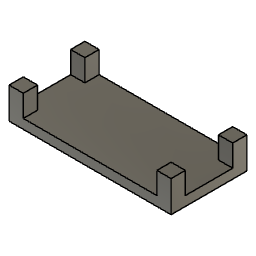
Reservoir Stand (Autodesk Fusion 360 design; units mm, degrees)
Autodesk Fusion 360 part; units mm, degrees
sketch "Sketch1" plane through (0, 0, 0) normal (0, 0, 1) x (1, 0, 0)
  line L0 (0, 0) -> (171, 0)
  line L1 (171, 0) -> (171, 80)
  line L2 (171, 80) -> (0, 80)
  line L3 (0, 80) -> (0, 0)
  dimension "d1" = 80
  dimension "d2" = 171
  constraint horizontal L0
  constraint vertical L1
  constraint horizontal L2
  constraint vertical L3
  constraint coincident L0.start L3.end
  measures "d1" distance of L0 L2
  measures "d2" distance of L1 L3
extrude "Extrude1" add sketch "Sketch1" along normal blind 7
sketch "Sketch2" plane through (0, 0, 7) normal (0, 0, 1) x (-1, 0, 0)
  line L0 (0, -80) -> (0, 0)
  line L1 (0, 0) -> (-171, 0)
  line L2 (-171, 0) -> (-171, -80)
  line L3 (-171, -80) -> (0, -80)
  line L4 (0, 0) -> (-15, 0)
  line L5 (-15, 0) -> (-15, -15)
  line L6 (-15, -15) -> (0, -15)
  line L7 (0, -15) -> (0, 0)
  line L8 (-85.5, 0) -> (-85.5, -80)
  line L9 (-156, 0) -> (-156, -15)
  line L10 (-156, -15) -> (-171, -15)
  line L11 (-171, -15) -> (-171, 0)
  line L12 (-171, 0) -> (-156, 0)
  line L13 (0, -40) -> (-171, -40)
  line L14 (-15, -65) -> (0, -65)
  line L15 (0, -65) -> (0, -80)
  line L16 (0, -80) -> (-15, -80)
  line L17 (-15, -80) -> (-15, -65)
  line L18 (-156, -80) -> (-156, -65)
  line L19 (-156, -65) -> (-171, -65)
  line L20 (-171, -65) -> (-171, -80)
  line L21 (-171, -80) -> (-156, -80)
  dimension "d5" = 15
  dimension "d6" = 15
  constraint horizontal L4
  constraint vertical L5
  constraint horizontal L6
  constraint vertical L7
  constraint coincident L0.end L1.start
  constraint midpoint L1 L8.start
  constraint midpoint L3 L8.end
  constraint symmetric L0.end L8 L1.end
  constraint symmetric L4.end L8 L9.start
  constraint symmetric L5.end L8 L9.end
  constraint symmetric L6.end L8 L10.end
  constraint midpoint L0 L13.start
  constraint midpoint L2 L13.end
  constraint symmetric L0.end L13 L0.start
  constraint symmetric L4.end L13 L16.end
  constraint symmetric L5.end L13 L14.start
  constraint symmetric L6.end L13 L14.end
  constraint symmetric L9.start L13 L18.start
  constraint symmetric L9.end L13 L18.end
  constraint symmetric L10.end L13 L19.end
  constraint symmetric L1.end L13 L2.end
  measures "d5" distance of L4 L6
  measures "d6" distance of L5 L7
extrude "Extrude2" add sketch "Sketch2" along normal blind 23 contours L0 L3 L14 L15 L16 L17 | L0 L1 L4 L5 L6 L7 | L2 L3 L18 L19 L20 L21 | L1 L2 L9 L10 L11 L12
sketch "Sketch3" plane through (0, 0, 0) normal (0, 0, -1) x (1, 0, 0)
  line L0 (0, 0) -> (0, -80)
  line L1 (0, -80) -> (171, -80)
  line L2 (171, -80) -> (171, 0)
  line L3 (171, 0) -> (0, 0)
  line L4 (166.5, -4.5) -> (4.5, -4.5)
  line L5 (4.5, -4.5) -> (4.5, -75.5)
  line L6 (4.5, -75.5) -> (166.5, -75.5)
  line L7 (166.5, -75.5) -> (166.5, -4.5)
  dimension "d9" = 4.5
  dimension "d10" = 4.5
  dimension "d11" = 4.5
  dimension "d12" = 4.5
  constraint horizontal L4
  constraint vertical L5
  constraint horizontal L6
  constraint vertical L7
  measures "d9" distance of L2 L7
  measures "d10" distance of L0 L5
  measures "d11" distance of L1 L6
  measures "d12" distance of L3 L4
extrude "Extrude3" add sketch "Sketch3" along normal blind 3
